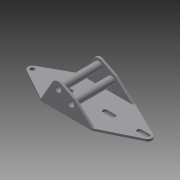
# Autodesk Inventor part: garage door hinge
Saved by Autodesk Inventor 2015 SP1 (Build 190203100, 203)
## iProperties
Created: 2015-01-12
Part Number: garage door hinge
Material: Generic
Document SubType Name: Modeling
Designer: Jarod
Density: 1 g/cm^3
Appearance: Default
Author: Jarod
Autodesk Inventor part; units mm, degrees
ref_plane "YZ Plane" through (0, 0, 0) normal (1, 0, 0) x (0, 1, 0)
ref_plane "XZ Plane" through (0, 0, 0) normal (0, 1, 0) x (-1, 0, 0)
ref_plane "XY Plane" through (0, 0, 0) normal (0, 0, 1) x (1, 0, 0)
sketch "Sketch1" plane through (0, 0, 0) normal (0, 1, 0) x (-1, 0, 0)
  line L0 (0, 0) -> (-76.2, 0)
  line L1 (-76.2, 0) -> (-76.2, -63.5) construction
  line L2 (-76.2, -63.5) -> (0, -63.5)
  line L3 (0, -63.5) -> (0, 0) construction
  line L4 (0, -31.75) -> (44.45, -31.75) construction
  line L5 (-76.2, -31.75) -> (-127, -31.75) construction
  circle A0 centre (44.45, -31.75) radius 3.175
  circle A1 centre (-127, -31.75) radius 3.175 construction
  circle A2 centre (-114.3, -31.75) radius 3.175 construction
  line L6 (-114.3, -34.925) -> (-127, -34.925)
  line L7 (-114.3, -28.575) -> (-127, -28.575)
  arc A3 (-114.3, -34.925) -> (-114.3, -28.575) centre (-114.3, -31.75) ccw
  arc A4 (-127, -28.575) -> (-127, -34.925) centre (-127, -31.75) ccw
  line L8 (0, -63.5) -> (47.5152, -37.3112)
  line L9 (47.5152, -26.1888) -> (0, 0)
  line L10 (-76.2, -63.5) -> (-129.7757, -37.4612)
  line L11 (-129.7757, -26.0388) -> (-76.2, 0)
  arc A5 (47.5152, -37.3112) -> (47.5152, -26.1888) centre (44.45, -31.75) ccw
  arc A6 (-129.7757, -26.0388) -> (-129.7757, -37.4612) centre (-127, -31.75) ccw
  circle A7 centre (-76.2, -31.75) radius 3.175 construction
  circle A8 centre (-63.5, -31.75) radius 3.175 construction
  line L12 (-76.2, -28.575) -> (-63.5, -28.575) construction
  line L13 (-76.2, -34.925) -> (-63.5, -34.925) construction
  line L14 (-63.5, -28.575) -> (-76.2, -28.575)
  line L15 (-76.2, -34.925) -> (-63.5, -34.925)
  arc A9 (-63.5, -34.925) -> (-63.5, -28.575) centre (-63.5, -31.75) ccw
  arc A10 (-76.2, -28.575) -> (-76.2, -34.925) centre (-76.2, -31.75) ccw
  circle A11 centre (0, -31.75) radius 3.175 construction
  circle A12 centre (-12.7, -31.75) radius 3.175 construction
  line L16 (0, -28.575) -> (-12.7, -28.575) construction
  line L17 (0, -34.925) -> (-12.7, -34.925) construction
  arc A13 (-12.7, -28.575) -> (-12.7, -34.925) centre (-12.7, -31.75) ccw
  arc A14 (0, -34.925) -> (0, -28.575) centre (0, -31.75) ccw
  line L18 (-12.7, -34.925) -> (0, -34.925)
  line L19 (-12.7, -28.575) -> (0, -28.575)
  dimension "d0" = 76.2
  dimension "d1" = 63.5
  dimension "d2" = 44.45
  dimension "d3" = 50.8
  dimension "d4" = 6.35
  dimension "d5" = 6.35
  dimension "d6" = 6.35
  dimension "d7" = 12.7
  dimension "d8" = 6.35
  dimension "d9" = 0
  dimension "d10" = 0
  dimension "d11" = 0
  dimension "d12" = 0
  dimension "d13" = 6.35
  dimension "d14" = 6.35
  dimension "d15" = 12.7
  dimension "d16" = 0
  dimension "d17" = 6.35
  dimension "d18" = 6.35
  dimension "d19" = 0
  dimension "d20" = 12.7
  constraints: 40 end point, 28 point on circle, 23 tangent, 15 centre point, 5 point on line, 4 coincident, 3 equal length, 3 horizontal, 2 equal radius, 2 midpoint, 1 perpendicular
  measures "d0" distance of L2.end L1.end
  measures "d1" distance of L1.end L0.end
  measures "d2" distance of L4.start L4.end
  measures "d3" distance of L5.start L5.end
  measures "d4" diameter of A0
  measures "d5" diameter of A1
  measures "d6" diameter of A2
  measures "d7" distance of L5.end A2.centre
  measures "d8" radius of A5
  measures "d9" distance of L4.end A5.centre
  measures "d10" distance of L4.end A5.centre
  measures "d11" distance of A4.centre A6.centre
  measures "d12" distance of L5.end A6.centre
  measures "d13" diameter of A7
  measures "d14" diameter of A8
  measures "d15" distance of L5.start A8.centre
  measures "d16" vertical distance of L5.start A8.centre
  measures "d17" diameter of A11
  measures "d18" diameter of A12
  measures "d19" vertical distance of L4.start A12.centre
  measures "d20" distance of L4.start A12.centre
extrude "Extrusion1" add sketch "Sketch1" along normal blind 3.175
sketch "Sketch2" plane through (0, 0, 0) normal (0, 0, 1) x (1, 0, 0)
  line L0 (0, 0) -> (76.2, 0) projected
  line L1 (76.2, 0) -> (76.2, 3.175) projected
  line L2 (0, 3.175) -> (76.2, 3.175) projected
  line L3 (0, 0) -> (0, 3.175) projected
  circle A0 centre (25.4, 28.575) radius 5.5562
  circle A1 centre (44.45, 19.05) radius 5.5563
  line L4 (0, 3.175) -> (17.12, 33.2832)
  line L5 (29.6597, 37.0944) -> (48.7097, 27.5694)
  line L6 (50.8395, 26.114) -> (76.2, 3.175)
  arc A2 (29.6597, 37.0944) -> (17.12, 33.2832) centre (25.4, 28.575) ccw
  arc A3 (50.8395, 26.114) -> (48.7097, 27.5694) centre (44.45, 19.05) ccw
  dimension "d23" = 11.1125
  dimension "d24" = 28.575
  dimension "d25" = 25.4
  dimension "d26" = 11.1125
  dimension "d27" = 19.05
  dimension "d28" = 31.75
  dimension "d29" = 9.525
  constraints: 6 end point, 4 centre point, 4 point on circle, 4 tangent, 2 coincident, 1 equal radius
  measures "d23" diameter of A0
  measures "d24" distance from line of L0 A0.centre
  measures "d25" horizontal distance of point (0, 0) A0.centre
  measures "d26" diameter of A1
  measures "d27" distance from line of L0 A1.centre
  measures "d28" distance from line of L1 A1.centre
  measures "d29" radius of A2
extrude "Extrusion2" add sketch "Sketch2" against normal blind 3.175
sketch "Sketch3" plane through (76.2, 0, -63.5) normal (0, 0, -1) x (-1, 0, 0)
  line L0 (0, 0) -> (76.2, 0) projected
  line L1 (76.2, 0) -> (76.2, 3.175) projected
  line L2 (0, 3.175) -> (76.2, 3.175) projected
  line L3 (0, 0) -> (0, 3.175) projected
  line L4 (76.2, 3.175) -> (0, 3.175) projected
  line L5 (76.2, 3.175) -> (59.08, 33.2832) projected
  arc A0 (59.08, 33.2832) -> (46.5403, 37.0944) centre (50.8, 28.575) ccw projected
  line L6 (46.5403, 37.0944) -> (27.4903, 27.5694) projected
  arc A1 (27.4903, 27.5694) -> (25.3605, 26.114) centre (31.75, 19.05) ccw projected
  line L7 (25.3605, 26.114) -> (0, 3.175) projected
  circle A2 centre (31.75, 19.05) radius 5.5563 projected
  circle A3 centre (50.8, 28.575) radius 5.5562 projected
  point P0 (76.2, 0)
extrude "Extrusion3" add sketch "Sketch3" against normal blind 3.175
sketch "Sketch4" plane through (0, 0, 0) normal (0, 0, 1) x (1, 0, 0)
  circle A0 centre (44.45, 19.05) radius 5.5563 projected
  circle A1 centre (25.4, 28.575) radius 5.5562 projected
  line L0 (0, 0) -> (76.2, 0) projected
  line L1 (76.2, 0) -> (76.2, 3.175) projected
  line L2 (76.2, 3.175) -> (50.8395, 26.114) projected
  arc A2 (50.8395, 26.114) -> (48.7097, 27.5694) centre (44.45, 19.05) ccw projected
  line L3 (48.7097, 27.5694) -> (29.6597, 37.0944) projected
  arc A3 (29.6597, 37.0944) -> (17.12, 33.2832) centre (25.4, 28.575) ccw projected
  line L4 (17.12, 33.2832) -> (0, 3.175) projected
  line L5 (0, 0) -> (0, 3.175) projected
  circle A4 centre (25.4, 28.575) radius 4.7625
  circle A5 centre (44.45, 19.05) radius 4.7625
  dimension "d34" = 9.525
  dimension "d35" = 9.525
  constraints: 2 centre point, 2 coincident
  measures "d34" diameter of A4
  measures "d35" diameter of A5
extrude "Extrusion4" add sketch "Sketch4" against normal blind 63.5 contours A0 | A1
body "Solid1"
